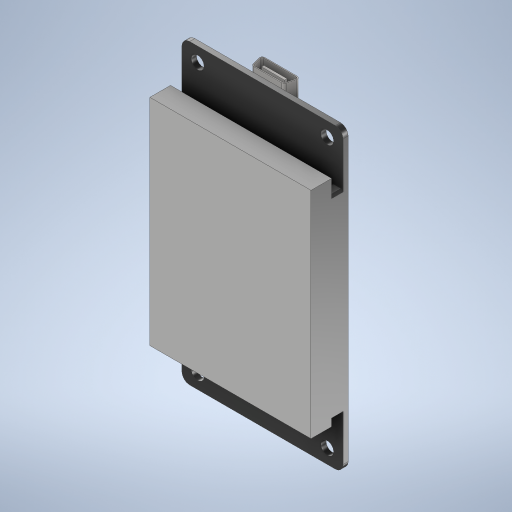
# Autodesk Inventor part: esp32s
Saved by Autodesk Inventor 2023 (Build 270158000, 158)
## iProperties
Created: 2022-06-15
Part Number: esp32s
Material: 일반
Document SubType Name: Modeling
Designer: user
Density: 1 g/cm^3
Appearance: 기본값
Author: user
Autodesk Inventor part; units mm, degrees
ref_plane "YZ Plane" through (0, 0, 0) normal (1, 0, 0) x (0, 1, 0)
ref_plane "XZ Plane" through (0, 0, 0) normal (0, 1, 0) x (-1, 0, 0)
ref_plane "XY Plane" through (0, 0, 0) normal (0, 0, 1) x (1, 0, 0)
sketch "스케치1" plane through (0, 0, 0) normal (0, 0, 1) x (1, 0, 0)
  line L0 (-14.1, 28.8) -> (14.1, 28.8)
  line L1 (15.6, 27.3) -> (15.6, -27.3)
  line L2 (14.1, -28.8) -> (-14.1, -28.8)
  line L3 (-15.6, -27.3) -> (-15.6, 27.3)
  line L4 (-15.6, 28.8) -> (15.6, -28.8) construction
  line L5 (15.6, 28.8) -> (-15.6, -28.8) construction
  circle A0 centre (-12.55, 26.05) radius 1.25
  line L6 (0, 0) -> (0, 13.0962) construction
  line L7 (0, 0) -> (6.3269, 0)
  circle A1 centre (12.55, 26.05) radius 1.25
  circle A2 centre (-12.55, -26.05) radius 1.25
  circle A3 centre (12.55, -26.05) radius 1.25
  arc A4 (-14.1, 28.8) -> (-15.6, 27.3) centre (-14.1, 27.3) ccw
  arc A5 (15.6, 27.3) -> (14.1, 28.8) centre (14.1, 27.3) ccw
  arc A6 (14.1, -28.8) -> (15.6, -27.3) centre (14.1, -27.3) ccw
  arc A7 (-15.6, -27.3) -> (-14.1, -28.8) centre (-14.1, -27.3) ccw
  dimension "d0" = 31.2
  dimension "d1" = 57.6
  dimension "d2" = 2.5
  dimension "d6" = 25.1
  dimension "d9" = 1.5
  dimension "d64" = 52.1
  constraints: 16 end point, 8 centre point, 8 point on circle, 8 point on line, 8 tangent, 3 equal radius, 3 symmetric about line, 2 midpoint, 2 parallel, 2 perpendicular, 1 horizontal, 1 vertical, 3 other
  measures "d0" distance of L4.end L5.end
  measures "d1" distance of L5.start L4.end
  measures "d2" diameter of A0
  measures "d6" distance of A1.centre A0.centre
  measures "d9" radius of A4
  measures "d64" distance of A2.centre A0.centre
extrude "돌출1" add sketch "스케치1" along normal blind 1
sketch "스케치2" plane through (-14.1, 28.8, 0) normal (0, 1, 0) x (1, 0, 0)
  line L0 (10.9516, 2.6) -> (17.2484, 2.6)
  line L1 (17.9, 2.6) -> (17.9, 0)
  line L2 (16.8197, 0) -> (11.3803, 0)
  line L3 (10.3, 0) -> (10.3, 2.6)
  line L4 (10.3, 2.6) -> (17.9, 0) construction
  line L5 (17.9, 2.6) -> (10.3, 0) construction
  line L6 (28.2, 0) -> (0, 0) projected
  line L7 (10.4686, 1.9706) -> (10.8974, 0.3706)
  line L8 (14.1, 1.3) -> (14.1, 2.6) construction
  line L9 (17.7314, 1.9706) -> (17.3026, 0.3706)
  arc A0 (10.9516, 2.6) -> (10.4686, 1.9706) centre (10.9516, 2.1) ccw
  arc A1 (17.7314, 1.9706) -> (17.2484, 2.6) centre (17.2484, 2.1) ccw
  arc A2 (16.8197, 0) -> (17.3026, 0.3706) centre (16.8197, 0.5) ccw
  arc A3 (10.8974, 0.3706) -> (11.3803, 0) centre (11.3803, 0.5) ccw
  line L10 (17.2484, 2.4) -> (10.9516, 2.4)
  arc A4 (10.9516, 2.4) -> (10.6618, 2.0224) centre (10.9516, 2.1) ccw
  line L11 (10.6618, 2.0224) -> (11.0906, 0.4224)
  arc A5 (11.0906, 0.4224) -> (11.3803, 0.2) centre (11.3803, 0.5) ccw
  line L12 (11.3803, 0.2) -> (16.8197, 0.2)
  arc A6 (16.8197, 0.2) -> (17.1094, 0.4224) centre (16.8197, 0.5) ccw
  line L13 (17.1094, 0.4224) -> (17.5382, 2.0224)
  arc A7 (17.5382, 2.0224) -> (17.2484, 2.4) centre (17.2484, 2.1) ccw
  point P0 (14.1, 0)
  point P1 (14.1, 0)
  point P2 (10.9967, 0)
  point P3 (17.2033, 0)
  dimension "d10" = 7.6
  dimension "d11" = 2.6
  dimension "d12" = 15
  dimension "d13" = 0.5
  dimension "d14" = 0.5
  dimension "d15" = 0.2
  constraints: 26 end point, 16 point on circle, 9 point on line, 8 centre point, 8 tangent, 5 midpoint, 3 parallel, 2 equal radius, 1 horizontal, 1 perpendicular, 1 symmetric about line, 7 other
  measures "d10" distance of L1.end L3.start
  measures "d11" distance of L1.start L1.end
  measures "d12" angle of L3 L7
  measures "d13" radius of A0
  measures "d14" radius of A1
  measures "d15" distance between parallel lines of L0 L10
extrude "돌출2" add sketch "스케치2" along normal blind 1 and the other way blind 5.6
sketch "스케치3" plane through (-14.1, 23.2, 0) normal (0, -1, 0) x (1, 0, 0)
  arc A0 (11.3803, 0) -> (10.8974, -0.3706) centre (11.3803, -0.5) ccw projected
  line L0 (10.8974, -0.3706) -> (10.4686, -1.9706) projected
  arc A1 (10.4686, -1.9706) -> (10.9516, -2.6) centre (10.9516, -2.1) ccw projected
  line L1 (10.9516, -2.6) -> (17.2484, -2.6) projected
  arc A2 (17.2484, -2.6) -> (17.7314, -1.9706) centre (17.2484, -2.1) ccw projected
  line L2 (17.7314, -1.9706) -> (17.3026, -0.3706) projected
  arc A3 (17.3026, -0.3706) -> (16.8197, 0) centre (16.8197, -0.5) ccw projected
  line L3 (11.3803, 0) -> (16.8197, 0) projected
  arc A4 (17.2484, -2.4) -> (17.5382, -2.0224) centre (17.2484, -2.1) ccw projected
  line L4 (17.2484, -2.4) -> (10.9516, -2.4) projected
  arc A5 (10.6618, -2.0224) -> (10.9516, -2.4) centre (10.9516, -2.1) ccw projected
  line L5 (10.6618, -2.0224) -> (11.0906, -0.4224) projected
  arc A6 (11.3803, -0.2) -> (11.0906, -0.4224) centre (11.3803, -0.5) ccw projected
  line L6 (11.3803, -0.2) -> (16.8197, -0.2) projected
  arc A7 (17.1094, -0.4224) -> (16.8197, -0.2) centre (16.8197, -0.5) ccw projected
  line L7 (17.1094, -0.4224) -> (17.5382, -2.0224) projected
  point P0 (14.1, 0)
extrude "돌출3" add sketch "스케치3" against normal blind 1 contours L4 A5 L5 A6 L6 A7 L7 A4
sketch "스케치4" plane through (-14.1, 24.2, 0) normal (0, 1, 0) x (1, 0, 0)
  line L0 (10.9516, 2.4) -> (17.2484, 2.4) projected
  arc A0 (10.9516, 2.4) -> (10.6618, 2.0224) centre (10.9516, 2.1) ccw projected
  line L1 (11.0906, 0.4224) -> (10.6618, 2.0224) projected
  arc A1 (11.0906, 0.4224) -> (11.3803, 0.2) centre (11.3803, 0.5) ccw projected
  line L2 (16.8197, 0.2) -> (11.3803, 0.2) projected
  arc A2 (16.8197, 0.2) -> (17.1094, 0.4224) centre (16.8197, 0.5) ccw projected
  line L3 (17.5382, 2.0224) -> (17.1094, 0.4224) projected
  arc A3 (17.5382, 2.0224) -> (17.2484, 2.4) centre (17.2484, 2.1) ccw projected
  line L4 (10.9516, 2.4) -> (17.2484, 2.4) projected
  line L5 (14.1, 2.4) -> (14.1, 0.2)
  line L6 (16.8197, 0.2) -> (11.3803, 0.2) projected
  line L7 (11.85, 1.05) -> (16.35, 1.05)
  line L8 (16.35, 1.05) -> (16.35, 1.55)
  line L9 (16.35, 1.55) -> (11.85, 1.55)
  line L10 (11.85, 1.55) -> (11.85, 1.05)
  line L11 (11.85, 1.05) -> (16.35, 1.55) construction
  line L12 (16.35, 1.05) -> (11.85, 1.55) construction
  point P0 (14.1, 0)
  point P1 (14.1, 1.3)
  dimension "d22" = 4.5
  dimension "d23" = 0.5
  constraints: 14 end point, 5 midpoint, 2 parallel, 1 horizontal, 1 perpendicular
  measures "d22" distance of L9.end L8.end
  measures "d23" distance of L8.end L7.end
extrude "돌출4" add sketch "스케치4" along normal blind 5.25 contours L9 L8 L7 L5 | L5 L7 L10 L9
sketch "스케치5" plane through (0, 0, 0) normal (0, 0, -1) x (-1, 0, 0)
  line L0 (8, -4.8) -> (-8, -4.8)
  line L1 (-8, -4.8) -> (-8, -28.8)
  line L2 (-8, -28.8) -> (8, -28.8)
  line L3 (8, -28.8) -> (8, -4.8)
  line L4 (8, -4.8) -> (-8, -28.8) construction
  line L5 (-8, -4.8) -> (8, -28.8) construction
  line L6 (14.1, -28.8) -> (-14.1, -28.8) projected
  line L7 (8, -20.8) -> (-8, -20.8)
  line L8 (-8, -20.8) -> (-8, -4.8)
  line L9 (-8, -4.8) -> (8, -4.8)
  line L10 (8, -4.8) -> (8, -20.8)
  line L11 (8, -20.8) -> (-8, -4.8) construction
  line L12 (-8, -20.8) -> (8, -4.8) construction
  line L13 (-7.8, -20.6) -> (7.8, -20.6)
  line L14 (7.8, -20.6) -> (7.8, -5)
  line L15 (7.8, -5) -> (-7.8, -5)
  line L16 (-7.8, -5) -> (-7.8, -20.6)
  point P0 (0, 0)
  point P1 (0, -16.8)
  point P2 (0, -12.8)
  point P3 (0, -4.8)
  point P4 (-8, -20.8)
  dimension "d26" = 24
  dimension "d27" = 16
  dimension "d28" = 16
  dimension "d49" = 0.2
  constraints: 32 end point, 6 midpoint, 6 parallel, 3 perpendicular, 3 point on line, 2 horizontal, 1 vertical alignment, 3 other
  measures "d26" distance of L0.end L1.end
  measures "d27" distance of L1.end L2.end
  measures "d28" distance between parallel lines of L9 L7
  measures "d49" distance between parallel lines of L7 L13
extrude "돌출5" add sketch "스케치5" along normal blind 0.66 contours L3 L7 L1 L0 | L3 L2 L1 L7 | L16 L15 L14 L13
extrude "돌출6" add sketch "스케치5" along normal blind 2.7 contours L16 L15 L14 L13
fillet "모깎기1" radius 0.2 2 edges at (8, -28.8, -0.33) (-8, -28.8, -0.33)
sketch "스케치6" plane through (0, 0, -0.66) normal (0, 0, -1) x (-1, 0, 0)
  line L0 (7.2056, -21.0177) -> (7.2056, -28.0434)
  line L1 (7.2056, -28.0434) -> (2.3744, -28.0434)
  line L2 (2.3744, -28.0434) -> (2.3744, -21.7967)
  line L3 (2.3744, -21.7967) -> (0.1881, -21.7967)
  line L4 (0.1881, -21.7967) -> (0.1881, -28.0434)
  line L5 (0.1881, -28.0434) -> (-3.1268, -28.0434)
  line L6 (-3.1268, -28.0434) -> (-3.1268, -21.7967)
  line L7 (-3.1268, -21.7967) -> (-5.0663, -21.7967)
  line L8 (-5.0663, -21.7967) -> (-5.0663, -28.0434)
  line L9 (-5.0663, -28.0434) -> (-7.3232, -28.0434)
  line L10 (-7.3232, -28.0434) -> (-7.3232, -20.9199)
  line L11 (8, -16) -> (-8, -16) construction
  line L12 (-6.8232, -20.9199) -> (-6.8232, -27.5434)
  line L13 (-6.8232, -27.5434) -> (-5.5663, -27.5434)
  line L14 (-5.5663, -27.5434) -> (-5.5663, -21.2967)
  line L15 (-5.5663, -21.2967) -> (-2.6268, -21.2967)
  line L16 (-2.6268, -21.2967) -> (-2.6268, -27.5434)
  line L17 (-2.6268, -27.5434) -> (-0.3119, -27.5434)
  line L18 (-0.3119, -27.5434) -> (-0.3119, -21.2967)
  line L19 (-0.3119, -21.2967) -> (2.8744, -21.2967)
  line L20 (2.8744, -21.2967) -> (2.8744, -27.5434)
  line L21 (2.8744, -27.5434) -> (6.7056, -27.5434)
  line L22 (6.7056, -27.5434) -> (6.7056, -21.0177)
  line L23 (7.2056, -21.0177) -> (6.7056, -21.0177)
  line L24 (-6.8232, -20.9199) -> (-7.3232, -20.9199)
  point P0 (0, 0)
  point P1 (7.8, -16)
  point P2 (-7.8, -16)
  dimension "d34" = 0.5
  constraints: 50 end point, 13 perpendicular, 6 point on line, 2 horizontal, 1 vertical, 10 other
  measures "d34" distance between parallel lines of L1 L21
extrude "돌출7" cut sketch "스케치6" against normal blind 0.1
sketch "스케치7" plane through (0, 0, 1) normal (0, 0, 1) x (1, 0, 0)
  line L0 (-15.2, 18.8) -> (-13.7, 18.8)
  line L1 (-13.3, 18.4) -> (-13.3, -18.4)
  line L2 (-13.7, -18.8) -> (-15.2, -18.8)
  line L3 (-15.6, -18.4) -> (-15.6, 18.4)
  line L4 (-15.6, 18.8) -> (-13.3, -18.8) construction
  line L5 (-13.3, 18.8) -> (-15.6, -18.8) construction
  line L6 (-15.6, 27.3) -> (-15.6, -27.3) projected
  line L7 (-13.7, 18.8) -> (-13.3, 18.4)
  line L8 (-15.2, 18.8) -> (-15.6, 18.4)
  line L9 (-13.3, -18.4) -> (-13.7, -18.8)
  line L10 (-15.2, -18.8) -> (-15.6, -18.4)
  point P0 (0, 0)
  point P1 (-14.45, 0)
  point P2 (-15.6, 0)
  dimension "d37" = 37.6
  dimension "d38" = 2.3
  dimension "d41" = 0.4
  dimension "d42" = 0.4
  dimension "d43" = 0.4
  dimension "d44" = 0.4
  dimension "d45" = 0.4
  dimension "d46" = 0.4
  dimension "d47" = 0.4
  dimension "d48" = 0.4
  constraints: 20 end point, 8 point on line, 4 midpoint, 2 parallel, 1 horizontal, 1 perpendicular
  measures "d37" distance of L5.start L4.end
  measures "d38" distance of L4.start L5.start
  measures "d41" distance of L0.end L5.start
  measures "d42" distance of L1.start L5.start
  measures "d43" distance of L0.start L4.start
  measures "d44" distance of L3.end L4.start
  measures "d45" distance of L1.end L4.end
  measures "d46" distance of L2.start L4.end
  measures "d47" distance of L2.end L5.end
  measures "d48" distance of L3.start L5.end
extrude "돌출8" add sketch "스케치7" along normal blind 2.2
mirror "미러1" about plane through (0, 0, 0) normal (1, 0, 0) of "돌출8"
fillet "모깎기2" radius 0.2 4 edges at (-7.8, -5, -1.68) (7.8, -5, -1.68) (-7.8, -20.6, -1.68) (7.8, -20.6, -1.68)
sketch "스케치10" plane through (0, 0, 3.2) normal (0, 0, 1) x (1, 0, 0)
  line L0 (-15.6, 27.3) -> (-15.6, -27.3) projected
  line L1 (15.6, -27.3) -> (15.6, -18.4) projected
  line L2 (-15.6, 21.7893) -> (15.6, 21.7893)
  line L3 (15.6, 21.7893) -> (15.6, -19.8525)
  line L4 (15.6, -19.8525) -> (-15.6, -19.8525)
  line L5 (-15.6, -19.8525) -> (-15.6, 21.7893)
  point P0 (0, 0)
  point P1 (-15.6, -19.8525)
  constraints: 8 end point, 2 parallel, 2 point on line, 1 horizontal, 1 perpendicular
extrude "돌출12" add sketch "스케치10" along normal blind 4
equation "\"d42\" = d41"
equation "\"d43\" = d41"
equation "\"d44\" = d43"
equation "\"d45\" = d41"
equation "\"d46\" = d45"
equation "\"d47\" = d41"
equation "\"d48\" = d47"
